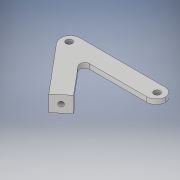
# Autodesk Inventor part: ventilador controladora_suportV
Saved by Autodesk Inventor 2019 (Build 230136000, 136)
## iProperties
Created: 2018-08-15
Part Number: ventilador controladora_suportV
Material: Genérico
Document SubType Name: Modeling
Designer: Albert Garangou Culebras
Density: 1 g/cm^3
Appearance: Valor por defecto
Author: Albert Garangou Culebras
Autodesk Inventor part; units mm, degrees
ref_plane "YZ Plane" through (0, 0, 0) normal (1, 0, 0) x (0, 1, 0)
ref_plane "XZ Plane" through (0, 0, 0) normal (0, 1, 0) x (-1, 0, 0)
ref_plane "XY Plane" through (0, 0, 0) normal (0, 0, 1) x (1, 0, 0)
sketch "Boceto1" plane through (0, 0, 0) normal (0, 1, 0) x (-1, 0, 0)
  line L0 (-2.031, 0) -> (-63, 0)
  line L1 (-65, -2) -> (-65, -8.0305)
  line L2 (-62.8998, -10.9676) -> (-2.0305, -10.9676)
  line L3 (0, -8.9987) -> (0, -2.031)
  line L4 (0, -8.9987) -> (0, -10.9676)
  line L5 (0, -10.9676) -> (-2.0305, -10.9676)
  line L6 (0, -2.031) -> (0, 0)
  line L7 (-65, -8.0305) -> (-65, -10.9676)
  line L8 (-65, -10.9676) -> (-62.8998, -10.9676)
  line L9 (-65, -2) -> (-65, 0)
  line L10 (-63, 0) -> (-65, 0)
  line L11 (0, 0) -> (-2.031, 0)
  dimension "d0" = 65
  constraints: 24 end point, 4 perpendicular, 4 point on line, 4 vertical, 3 horizontal
  measures "d0" distance of L6.end L9.end
extrude "Extrusión1" add sketch "Boceto1" along normal blind 3
sketch "Boceto2" plane through (0, 3, 0) normal (0, 1, 0) x (1, 0, 0)
  line L0 (0, 10.9676) -> (0, 0) projected
  circle A0 centre (5, 5.4838) radius 2
  line L1 (65, 0) -> (65, 10.9676) projected
  circle A1 centre (60, 5.4838) radius 2
  line L2 (65, 5.4838) -> (60, 5.4838)
  line L3 (0, 5.4838) -> (5, 5.4838)
  point P0 (0.1384, 8.9976)
  point P1 (0.0312, 2.0308)
  point P2 (65, 2)
  point P3 (65, 8.0305)
  dimension "d20" = 5
  dimension "d31" = 4
  dimension "d32" = 4
  constraints: 4 end point, 2 centre point, 2 horizontal, 1 coincident, 1 midpoint, 2 other
  measures "d20" distance of L2.start L2.end
  measures "d31" diameter of A0
  measures "d32" diameter of A1
extrude "Extrusión2" cut sketch "Boceto2" against normal blind 5
sketch "Boceto3" plane through (0, 3, 0) normal (0, 1, 0) x (1, 0, 0)
  circle A0 centre (5, 5.4838) radius 2 projected
  line L0 (5, 5.4838) -> (319.2562, 5.4838) construction
  line L1 (16.8683, -0.0721) -> (35.3706, -22.1223)
  line L2 (16.8683, -0.0721) -> (16.8078, 0)
  line L3 (8.4418, -7.1428) -> (2.4483, 0)
  line L4 (65, 0) -> (0, 0) projected
  line L5 (8.4418, -7.1428) -> (26.9441, -29.1929)
  line L6 (35.3706, -22.1223) -> (26.9441, -29.1929)
  constraints: 12 end point, 1 horizontal, 1 perpendicular, 1 point on line
extrude "Extrusión3" add sketch "Boceto3" against normal blind 3 contours L1 L6 L5 L3 L4 L2
sketch "Boceto4" plane through (0, 3, 0) normal (0, 1, 0) x (1, 0, 0)
  line L0 (0, 0) -> (2.4483, 0) projected
  line L1 (2.4483, 0) -> (0, 3)
  line L2 (0, 10.9676) -> (0, 0) projected
  line L3 (0, 3) -> (0, 0)
  line L4 (2.4483, 0) -> (0, 0)
  constraints: 6 end point, 2 collinear, 1 point on line
extrude "Extrusión4" cut sketch "Boceto4" against normal blind 15.5
fillet "Empalme2" [suppressed]
fillet "Empalme3" radius 3 1 edges at (16.8078, 1.5, 0)
sketch "Boceto5" plane through (0, 0, 0) normal (0, -1, 0) x (1, 0, 0)
  line L0 (35.3706, 22.1223) -> (26.9441, 29.1929) projected
  line L1 (35.3706, 22.1223) -> (26.9441, 29.1929)
  line L2 (26.9441, 29.1929) -> (23.7301, 25.3627)
  line L3 (26.9441, 29.1929) -> (2.4483, 0) projected
  line L4 (23.7301, 25.3627) -> (32.1566, 18.292)
  line L5 (20.9432, 4.9284) -> (35.3706, 22.1223) projected
  line L6 (32.1566, 18.292) -> (35.3706, 22.1223)
  line L7 (35.3706, 22.1223) -> (26.9441, 29.1929)
  point P0 (0, 0)
  dimension "d24" = 5
  constraints: 10 end point, 3 collinear, 2 point on line
  measures "d24" distance of L0.end L2.end
extrude "Extrusión5" add sketch "Boceto5" along normal blind 7
sketch "Boceto6" plane through (26.9441, -7, 29.1929) normal (0.6427876, 0, 0.7660444) x (0.7660444, 0, -0.6427876)
  line L0 (3.4796, 10) -> (7.4796, 10) projected
  line L1 (5.4796, 10) -> (5.4796, 5)
  circle A0 centre (5.4796, 5) radius 1.5
  point P0 (-1.8755, 7)
  dimension "d27" = 5
  dimension "d28" = 3
  constraints: 2 end point, 1 centre point, 1 coincident, 1 midpoint, 1 vertical
  measures "d27" distance of L1.start L1.end
  measures "d28" diameter of A0
extrude "Extrusión6" cut sketch "Boceto6" against normal blind 16.75
fillet "Empalme4" radius 5.5 1 edges at (65, 1.5, -10.9676)
fillet "Empalme5" radius 9 1 edges at (0, 1.5, -3)
fillet "Empalme6" radius 6 1 edges at (0, 1.5, -10.9676)
fillet "Empalme7" radius 6 1 edges at (65, 1.5, 0)
